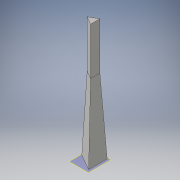
# Autodesk Inventor part: pillar
Saved by Autodesk Inventor 2016 (Build 200138000, 138)
## iProperties
Created: 2015-12-05
Part Number: pillar
Material: Generic
Document SubType Name: Modeling
Designer: acd
Density: 1 g/cm^3
Appearance: Default
Author: acd
Autodesk Inventor part; units mm, degrees
sketch "Sketch1" plane through (0, 0, 0) normal (0, 1, 0) x (-1, 0, 0)
  line L0 (11.7617, 136.6037) -> (11.7617, -163.3963)
  line L1 (11.7617, -163.3963) -> (271.5693, -13.3963)
  line L2 (271.5693, -13.3963) -> (11.7617, 136.6037)
  circle A0 centre (98.3643, -13.3963) radius 86.6025
  line L3 (55.063, 61.6037) -> (55.063, -88.3963)
  line L4 (55.063, 61.6037) -> (184.9668, -13.3963)
  line L5 (55.063, 61.6037) -> (205.063, 61.6037) construction
  line L6 (184.9668, -13.3963) -> (55.063, -88.3963)
  circle A1 centre (98.3643, -13.3963) radius 43.3013
  point P0 (85.0813, -150)
  point P1 (141.6655, 61.6037)
  point P2 (141.6655, -88.3963)
  point P3 (11.7617, -13.3963)
  point P4 (203.5969, -52.6402)
  dimension "d10" = 300
  dimension "d11" = 300
  dimension "d12" = 60
  dimension "d13" = 150
  dimension "d14" = 150
  dimension "d15" = 30
  constraints: 14 end point, 6 tangent, 3 midpoint, 2 centre point, 2 coincident, 2 vertical, 1 concentric, 1 equal length, 1 horizontal, 1 point on line
  measures "d10" distance of L0.start L0.end
  measures "d11" distance of L0.end L1.end
  measures "d12" angle of L1 L0
  measures "d13" distance of L3.start L3.end
  measures "d14" distance of L3.start L4.end
  measures "d15" angle of L4 L5
ref_plane "Work Plane1" through (-52.1275, 0, 74.1452) normal (0, -1, 0) x (0, 0, -1)
extrude "Extrusion2" add sketch "Sketch1" along normal blind 1219.2
sketch "Sketch2" plane through (0, 1219.2, 0) normal (0, 1, 0) x (1, 0, 0)
  line L0 (-271.5693, 13.3963) -> (-11.7617, -136.6037) projected
  line L1 (-11.7617, -136.6037) -> (-11.7617, 163.3963) projected
  line L2 (-11.7617, 163.3963) -> (-271.5693, 13.3963) projected
  circle A0 centre (-98.3643, 13.3963) radius 86.6025
  line L3 (-55.063, -61.6037) -> (-55.063, 88.3963)
  line L4 (-55.063, 88.3963) -> (-184.9668, 13.3963)
  line L5 (-184.9668, 13.3963) -> (-55.063, -61.6037)
  circle A1 centre (-98.3643, 13.3963) radius 43.3013
  point P0 (0, 0)
  point P1 (-141.6655, -61.6037)
  point P2 (-11.7617, 13.3963)
  point P3 (-141.6655, 88.3963)
  dimension "d18" = 150
  dimension "d19" = 150
  constraints: 6 end point, 6 tangent, 3 midpoint, 2 centre point, 1 concentric, 1 horizontal alignment, 1 vertical
  measures "d18" distance of L3.start L3.end
  measures "d19" distance of L3.end L4.end
ref_plane "Work Plane2" through (-55.063, 1219.2, 61.6037) normal (-0.9994, -0.0355, 0) x (0, 0, -1)
split "Split1" plane through (-55.063, 1219.2, 61.6037) removes the side toward (0.9994, 0.0355, 0)
ref_plane "Work Plane3" through (-184.9668, 1219.2, -13.3963) normal (0.4997, -0.0355, -0.8655) x (0.866, 0, 0.5)
split "Split2" plane through (-184.9668, 1219.2, -13.3963) removes the side toward (-0.4997, 0.0355, 0.8655)
ref_plane "Work Plane4" through (-55.063, 1219.2, -88.3963) normal (0.4997, -0.0355, 0.8655) x (-0.866, 0, 0.5)
split "Split3" plane through (-55.063, 1219.2, -88.3963) removes the side toward (-0.4997, 0.0355, -0.8655)
extrude "Extrusion3" add sketch "Sketch2" along normal blind 762 contours L4 A1 L5 | L5 A1 L3 | L3 A1 L4 | A1
body "Solid2"
